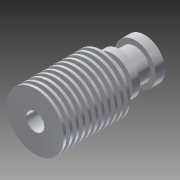
# Autodesk Inventor part: E3DV6HeatSink
Saved by Autodesk Inventor 2015 (Build 190159000, 159)
## iProperties
Created: 2014-08-17
Part Number: E3DV6HeatSink
Material: Aluminum 6061
Document SubType Name: Modeling
Designer: Jack
Density: 2.7 g/cm^3
Appearance: Aluminum - Flat
Author: Jack
Autodesk Inventor part; units mm, degrees
ref_plane "YZ Plane" through (0, 0, 0) normal (1, 0, 0) x (0, 1, 0)
ref_plane "XZ Plane" through (0, 0, 0) normal (0, 1, 0) x (-1, 0, 0)
ref_plane "XY Plane" through (0, 0, 0) normal (0, 0, 1) x (1, 0, 0)
sketch "Sketch1" plane through (0, 0, 0) normal (0, 0, 1) x (1, 0, 0)
  line L0 (0, 0) -> (-11.15, 0)
  line L1 (-11.15, 0) -> (-11.15, 1)
  line L2 (-11.15, 1) -> (0, 1)
  line L3 (0, 1) -> (0, 2.5)
  line L4 (0, 2.5) -> (-11.15, 2.5)
  line L5 (-11.15, 2.5) -> (-11.15, 3.5)
  line L6 (-11.15, 3.5) -> (0, 3.5)
  line L7 (0, 3.5) -> (0, 5)
  line L8 (0, 5) -> (-11.15, 5)
  line L9 (-11.15, 5) -> (-11.15, 6)
  line L10 (-11.15, 6) -> (0, 6)
  line L11 (0, 6) -> (0, 7.5)
  line L12 (0, 7.5) -> (-11.15, 7.5)
  line L13 (-11.15, 7.5) -> (-11.15, 8.5)
  line L14 (-11.15, 8.5) -> (0, 8.5)
  line L15 (0, 8.5) -> (0, 10)
  line L16 (0, 10) -> (-11.15, 10)
  line L17 (-11.15, 10) -> (-11.15, 11)
  line L18 (-11.15, 11) -> (0, 11)
  line L19 (0, 11) -> (0, 12.5)
  line L20 (0, 12.5) -> (-11.15, 12.5)
  line L21 (-11.15, 12.5) -> (-11.15, 13.5)
  line L22 (-11.15, 13.5) -> (0, 13.5)
  line L23 (0, 13.5) -> (0, 15)
  line L24 (0, 15) -> (-11.15, 15)
  line L25 (-11.15, 15) -> (-11.15, 16)
  line L26 (-11.15, 16) -> (0, 16)
  line L27 (0, 16) -> (0, 17.5)
  line L28 (0, 17.5) -> (-11.15, 17.5)
  line L29 (-11.15, 17.5) -> (-11.15, 18.5)
  line L30 (-11.15, 18.5) -> (0, 18.5)
  line L31 (0, 18.5) -> (0, 20)
  line L32 (0, 20) -> (-11.15, 20)
  line L33 (-11.15, 20) -> (-11.15, 21)
  line L34 (-11.15, 21) -> (0, 21)
  line L35 (0, 21) -> (0, 22.5)
  line L36 (0, 22.5) -> (-11.15, 22.5)
  line L37 (-11.15, 22.5) -> (-11.15, 23.5)
  line L38 (-11.15, 23.5) -> (0, 23.5)
  line L39 (0, 23.5) -> (0, 25)
  line L40 (0, 25) -> (-11.15, 25)
  line L41 (-11.15, 25) -> (-11.15, 26)
  line L42 (-11.15, 26) -> (0, 26)
  line L43 (0, 26) -> (0, 27.5)
  line L44 (0, 27.5) -> (-8, 27.5)
  line L45 (-8, 27.5) -> (-8, 28.5)
  line L46 (-8, 28.5) -> (0, 28.5)
  line L47 (0, 28.5) -> (0, 27.5)
  line L48 (0, 26) -> (0, 25)
  line L49 (0, 23.5) -> (0, 22.5)
  line L50 (0, 21) -> (0, 20)
  line L51 (0, 18.5) -> (0, 17.5)
  line L52 (0, 16) -> (0, 15)
  line L53 (0, 13.5) -> (0, 12.5)
  line L54 (0, 11) -> (0, 10)
  line L55 (0, 8.5) -> (0, 7.5)
  line L56 (0, 6) -> (0, 5)
  line L57 (0, 3.5) -> (0, 2.5)
  line L58 (0, 1) -> (0, 0)
  dimension "d0" = 11.15
  dimension "d1" = 1
  dimension "d2" = 1.5
  dimension "d3" = 8
  dimension "d4" = 1
  constraints: 118 end point, 36 point on line, 31 collinear, 28 perpendicular, 10 vertical alignment, 2 vertical, 1 horizontal
  measures "d0" distance of L0.start L0.end
  measures "d1" distance of L0.end L1.end
  measures "d2" distance of L2.end L3.end
  measures "d3" distance of L45.end L46.end
  measures "d4" distance of L44.end L45.end
revolve "Fins" add sketch "Sketch1" angle 360 about axis through (0, 23.5, 0) along (0, 1, 0)
sketch "Sketch3" plane through (0, 0, 0) normal (1, 0, 0) x (0, 1, 0)
  line L0 (0, 0) -> (0, 7)
  line L1 (0, -11.15) -> (0, 11.15) projected
  line L2 (30, 5) -> (30, 8)
  line L3 (0, 7) -> (30, 5)
  line L4 (28.5, -8) -> (28.5, 8) projected
  line L5 (30, 8) -> (33, 8)
  line L6 (33, 8) -> (33, 6)
  line L7 (33, 6) -> (39, 6)
  line L8 (39, 6) -> (39, 8)
  line L9 (39, 8) -> (42.7, 8)
  line L10 (42.7, 8) -> (42.7, 0)
  line L11 (42.7, 0) -> (0, 0)
  dimension "d20" = 7
  dimension "d21" = 8
  dimension "d22" = 5
  dimension "d23" = 1.5
  dimension "d24" = 3
  dimension "d25" = 6
  dimension "d26" = 6
  dimension "d27" = 3.7
  constraints: 20 end point, 3 horizontal, 3 perpendicular, 2 vertical, 1 horizontal alignment, 1 point on line
  measures "d20" distance of L0.start L0.end
  measures "d21" vertical distance of L0.start L2.end
  measures "d22" vertical distance of L0.start L2.start
  measures "d23" distance between parallel lines of L4 L2
  measures "d24" distance of L2.end L5.end
  measures "d25" vertical distance of L0.start L6.end
  measures "d26" distance of L6.end L7.end
  measures "d27" distance of L8.end L9.end
revolve "Body" add sketch "Sketch3" angle 360 about axis through (0, 42.7, 0) along (0, -1, 0)
sketch "Sketch4" plane through (0, 42.7, 0) normal (0, 1, 0) x (1, 0, 0)
  circle A0 centre (0, 0) radius 8 projected
  circle A1 centre (0, 0) radius 4
  dimension "d29" = 8
  constraints: 1 centre point, 1 coincident
  measures "d29" diameter of A1
extrude "CouplerHole" cut sketch "Sketch4" against normal blind 8 contours A1
sketch "Sketch5" plane through (0, 0, 0) normal (0, -1, 0) x (1, 0, 0)
  circle A0 centre (0, 0) radius 6.4333 projected
  circle A1 centre (0, 0) radius 3.5
  dimension "d32" = 7
  constraints: 1 centre point, 1 coincident
  measures "d32" diameter of A1
extrude "HeadBoltHole" cut sketch "Sketch5" against normal blind 10.5 contours A1
sketch "Sketch6" plane through (0, 10.5, 0) normal (0, -1, 0) x (1, 0, 0)
  circle A0 centre (0, 0) radius 3.5 projected
  circle A1 centre (0, 0) radius 2.1
  dimension "d35" = 4.2
  constraints: 1 centre point, 1 coincident
  measures "d35" diameter of A1
extrude "TubeHole" cut sketch "Sketch6" against normal up to surface (32.2 mm away) contours A1
body "Solid1"
